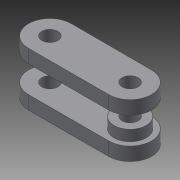
# Autodesk Inventor part: joint
Saved by Autodesk Inventor 2018 (Build 220112000, 112)
## iProperties
Created: 2019-02-20
Part Number: joint
Material: 一般
Document SubType Name: Modeling
Designer: ku_sk
Density: 1 g/cm^3
Appearance: 既定
Author: ku_sk
Autodesk Inventor part; units mm, degrees
ref_plane "YZ Plane" through (0, 0, 0) normal (1, 0, 0) x (0, 1, 0)
ref_plane "XZ Plane" through (0, 0, 0) normal (0, 1, 0) x (-1, 0, 0)
ref_plane "XY Plane" through (0, 0, 0) normal (0, 0, 1) x (1, 0, 0)
sketch "スケッチ1" plane through (0, 0, 0) normal (0, 0, 1) x (1, 0, 0)
  line L0 (-7.5, 0) -> (7.5, 0) construction
  line L1 (-7.5, -4) -> (7.5, -4)
  line L2 (7.5, 4) -> (-7.5, 4)
  arc A0 (-7.5, 4) -> (-7.5, -4) centre (-7.5, 0) ccw
  arc A1 (7.5, -4) -> (7.5, 4) centre (7.5, 0) ccw
  point P0 (0, 0)
  point P1 (0, 0)
  dimension "d0" = 4
  dimension "d1" = 15
  constraints: 8 end point, 4 point on circle, 4 tangent, 2 centre point, 1 coincident, 1 horizontal, 1 midpoint, 1 parallel
  measures "d0" radius of A1
  measures "d1" distance of L0.start L0.end
extrude "押し出し1" add sketch "スケッチ1" along normal mid plane 10
sketch "スケッチ2" plane through (0, 0, 0) normal (0, 0, 1) x (1, 0, 0)
  line L0 (7.5, -4) -> (-7.5, -4) projected
  arc A0 (-7.5, 4) -> (-7.5, -4) centre (-7.5, 0) ccw projected
  line L1 (-7.5, 4) -> (7.5, 4) projected
  arc A1 (7.5, -4) -> (7.5, 4) centre (7.5, 0) ccw projected
  point P0 (0, 0)
extrude "押し出し2" cut sketch "スケッチ2" along normal mid plane 5
sketch "スケッチ3" plane through (0, 0, 0) normal (0, 0, 1) x (1, 0, 0)
  circle A0 centre (-7.5, 0) radius 1.5
  circle A1 centre (7.5, 0) radius 1.5
  arc A2 (-7.5, 4) -> (-7.5, -4) centre (-7.5, 0) ccw projected
  arc A3 (7.5, -4) -> (7.5, 4) centre (7.5, 0) ccw projected
  point P0 (0, 0)
  dimension "d6" = 3
  dimension "d7" = 3
  constraints: 2 centre point, 2 concentric
  measures "d6" diameter of A0
  measures "d7" diameter of A1
extrude "押し出し3" cut sketch "スケッチ3" along normal through all both and the other way through all
sketch "スケッチ4" plane through (0, 0, -2.5) normal (0, 0, 1) x (1, 0, 0)
  circle A0 centre (7.5, 0) radius 1.5 projected
  circle A1 centre (7.5, 0) radius 3
  point P0 (0, 0)
  dimension "d10" = 1.5
  constraints: 1 centre point
  measures "d10" radial gap between concentric circles of A1 A0
extrude "押し出し4" add sketch "スケッチ4" along normal blind 2
